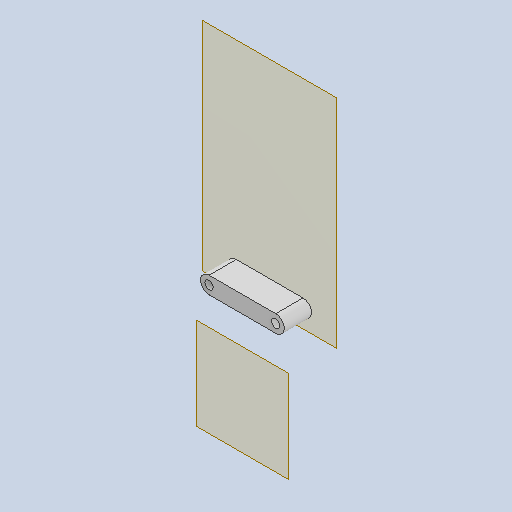
# Autodesk Inventor part: _thigh
Saved by Autodesk Inventor 2024.3 (Build 283343000, 343)
## iProperties
Created: 2024-09-06
Part Number: _thigh
Material: 일반
Document SubType Name: Modeling
Designer: gretc
Density: 1 g/cm^3
Appearance: 기본값
Author: gretc
Autodesk Inventor part; units mm, degrees
ref_plane "YZ Plane" through (0, 0, 0) normal (1, 0, 0) x (0, 1, 0)
ref_plane "XZ Plane" through (0, 0, 0) normal (0, 1, 0) x (-1, 0, 0)
ref_plane "XY Plane" through (0, 0, 0) normal (0, 0, 1) x (1, 0, 0)
ref_plane "작업 평면1" through (0, 0, 0) normal (0, 0, 1) x (1, 0, 0)
sketch "스케치1" plane through (0, 0, 0) normal (0, 0, 1) x (1, 0, 0)
  line L0 (13.5, -39.75) -> (11.5, -39.75) projected
  arc A0 (11.5, -39.75) -> (9.25, -42) centre (11.5, -42) ccw projected
  line L1 (9.25, -42) -> (9.25, -44) projected
  arc A1 (8.25, -45) -> (9.25, -44) centre (8.25, -44) ccw projected
  line L2 (8.25, -45) -> (-8.25, -45) projected
  arc A2 (-9.25, -44) -> (-8.25, -45) centre (-8.25, -44) ccw projected
  line L3 (-9.25, -44) -> (-9.25, -42) projected
  arc A3 (-9.25, -42) -> (-11.5, -39.75) centre (-11.5, -42) ccw projected
  line L4 (-11.5, -39.75) -> (-13.5, -39.75) projected
  arc A4 (-14.5, -38.75) -> (-13.5, -39.75) centre (-13.5, -38.75) ccw projected
  line L5 (-14.5, -38.75) -> (-14.5, 8.25) projected
  arc A5 (-13.5, 9.25) -> (-14.5, 8.25) centre (-13.5, 8.25) ccw projected
  line L6 (-13.5, 9.25) -> (-11.5, 9.25) projected
  arc A6 (-11.5, 9.25) -> (-9.25, 11.5) centre (-11.5, 11.5) ccw projected
  line L7 (-9.25, 11.5) -> (-9.25, 14.5) projected
  line L8 (-15, 14.5) -> (-9.25, 14.5) projected
  line L9 (-20.1, 8.5) -> (-15, 14.5) projected
  line L10 (-20.1, -44.6) -> (-20.1, 8.5) projected
  line L11 (-15, -50.6) -> (-20.1, -44.6) projected
  line L12 (15, -50.6) -> (-15, -50.6) projected
  line L13 (20.1, -44.6) -> (15, -50.6) projected
  line L14 (20.1, 8.5) -> (20.1, -44.6) projected
  line L15 (15, 14.5) -> (20.1, 8.5) projected
  line L16 (9.25, 14.5) -> (15, 14.5) projected
  line L17 (9.25, 14.5) -> (9.25, 11.5) projected
  arc A7 (9.25, 11.5) -> (11.5, 9.25) centre (11.5, 11.5) ccw projected
  line L18 (11.5, 9.25) -> (13.5, 9.25) projected
  arc A8 (14.5, 8.25) -> (13.5, 9.25) centre (13.5, 8.25) ccw projected
  line L19 (14.5, 8.25) -> (14.5, -38.75) projected
  arc A9 (13.5, -39.75) -> (14.5, -38.75) centre (13.5, -38.75) ccw projected
  circle A10 centre (17.3, 4) radius 1.35 projected
  circle A11 centre (17.3, -18) radius 1.35 projected
  circle A12 centre (11, -47.8) radius 1.35 projected
  circle A13 centre (-17.3, 4) radius 1.35 projected
  circle A14 centre (-17.3, -18) radius 1.35 projected
  circle A15 centre (-11, -47.8) radius 1.35 projected
  circle A16 centre (17.3, -40) radius 1.35 projected
  circle A17 centre (-17.3, -40) radius 1.35 projected
  line L20 (-10.8997, -45) -> (-7.025, -45) projected
  line L21 (-12.5, -45) -> (-11.1003, -45) projected
  line L22 (15, -50.6) -> (-15, -50.6) projected
  line L23 (11.1003, -45) -> (12.5, -45) projected
  line L24 (7.025, -45) -> (10.8997, -45) projected
  arc A18 (12.5, -45) -> (14.5, -43) centre (12.5, -43) ccw projected
  arc A19 (-14.5, -43) -> (-12.5, -45) centre (-12.5, -43) ccw projected
  circle A20 centre (-11, -47.8) radius 2.8
  circle A21 centre (11, -47.8) radius 2.8
  line L25 (15, -50.6) -> (-15, -50.6) projected
  line L26 (-10.8997, -45) -> (-7.025, -45) projected
  line L27 (8.25, -45) -> (-8.25, -45) projected
  line L28 (7.025, -45) -> (10.8997, -45) projected
  line L29 (15, -50.6) -> (-15, -50.6) projected
  line L30 (-11, -47.8) -> (11, -47.8)
  line L31 (11, -45) -> (-11, -45)
  line L32 (-11, -45) -> (-11, -50.6)
  line L33 (-11, -50.6) -> (11, -50.6)
  line L34 (11, -50.6) -> (11, -45)
  line L35 (11, -45) -> (-11, -50.6) construction
  line L36 (-11, -45) -> (11, -50.6) construction
  point P0 (0, 0)
  point P1 (0, -47.8)
  point P2 (-11, -50.6)
  point P3 (11, -50.6)
  point P4 (10.8997, -45)
  constraints: 14 end point, 3 midpoint, 3 parallel, 2 centre point, 2 coincident, 2 tangent, 1 horizontal, 1 perpendicular
extrude "돌출1" add sketch "스케치1" along normal blind 9 contours L24 A21 L30 A20 L20 L2 | A21 L34 A12 L30 | A21 L34 A12 | L30 A12 L34 A21 | A21 L12 A20 L30 | L30 A15 L32 A20 | A20 L32 A15 L30 | A20 L32 A15
ref_plane "작업 평면2" through (0, -75.1, 9) normal (0, 0, 1) x (1, 0, 0)
